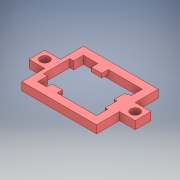
# Autodesk Inventor part: TP4056_long_holder
Saved by Autodesk Inventor 2018 (Build 220112000, 112)
## iProperties
Created: 2019-09-05
Part Number: TP4056_long_holder
Material: Generic
Document SubType Name: Modeling
Designer: ZEUSLAP
Density: 1 g/cm^3
Appearance: Default
Author: ZEUSLAP
## iProperties of the stored document charger_holder_TP4056_3DPrint.ipt
Created: 2019-10-07
Part Number: charger_holder_TP4056_3DPrint
Material: Generic
Document SubType Name: Modeling
Designer: ZEUSLAP
Density: 1 g/cm^3
Appearance: Default
Author: ZEUSLAP
Autodesk Inventor part; units mm, degrees
ref_plane "YZ Plane" through (0, 0, 0) normal (1, 0, 0) x (0, 1, 0)
ref_plane "XZ Plane" through (0, 0, 0) normal (0, 1, 0) x (-1, 0, 0)
ref_plane "XY Plane" through (0, 0, 0) normal (0, 0, 1) x (1, 0, 0)
sketch "shape" plane through (0, 0, 0) normal (0, 0, 1) x (1, 0, 0)
  line L0 (-11.25, 8.75) -> (11.25, 8.75)
  line L1 (11.25, 8.75) -> (11.25, -8.75)
  line L2 (11.25, -8.75) -> (-11.25, -8.75)
  line L3 (-11.25, -8.75) -> (-11.25, 8.75)
  line L4 (14.25, 11.75) -> (-14.25, 11.75)
  line L5 (-14.25, 11.75) -> (-14.25, -11.75)
  line L6 (-14.25, -11.75) -> (14.25, -11.75)
  line L7 (14.25, -11.75) -> (14.25, 11.75)
  line L8 (-12.75, 5) -> (-11.25, 5)
  line L9 (-11.25, 5) -> (-11.25, -5)
  line L10 (-11.25, -5) -> (-12.75, -5)
  line L11 (-12.75, -5) -> (-12.75, 5)
  line L12 (-7.75, -6.75) -> (-3.75, -6.75)
  line L13 (-3.75, -6.75) -> (-3.75, -8.75)
  line L14 (-3.75, -8.75) -> (-7.75, -8.75)
  line L15 (-7.75, -8.75) -> (-7.75, -6.75)
  line L16 (10.25, 4.5) -> (11.25, 4.5)
  line L17 (11.25, 4.5) -> (11.25, -4.5)
  line L18 (11.25, -4.5) -> (10.25, -4.5)
  line L19 (10.25, -4.5) -> (10.25, 4.5)
  line L20 (10.25, 1.5) -> (10.25, -1.5)
  line L21 (-5.75, 8.75) -> (-1.75, 8.75)
  line L22 (-1.75, 8.75) -> (-1.75, 6.25)
  line L23 (-1.75, 6.25) -> (-5.75, 6.25)
  line L24 (-5.75, 6.25) -> (-5.75, 8.75)
  line L25 (-20.25, 3) -> (-14.25, 3)
  line L26 (-14.25, 3) -> (-14.25, -3)
  line L27 (-14.25, -3) -> (-20.25, -3)
  line L28 (-20.25, -3) -> (-20.25, 3)
  line L29 (14.25, 3) -> (20.25, 3)
  line L30 (20.25, 3) -> (20.25, -3)
  line L31 (20.25, -3) -> (14.25, -3)
  line L32 (14.25, -3) -> (14.25, 3)
  circle A0 centre (-17.25, 0) radius 1.75
  circle A1 centre (17.25, 0) radius 1.75
  line L33 (9.25, 4) -> (10.25, 4)
  line L34 (10.25, 4) -> (10.25, 0)
  line L35 (10.25, 0) -> (9.25, 0)
  line L36 (9.25, 0) -> (9.25, 4)
  point P0 (0, 0)
  point P1 (0, 8.75)
  point P2 (11.25, 0)
  point P3 (-12.75, 0)
  point P4 (10.25, 0)
  point P5 (-14.25, 0)
  point P6 (14.25, 0)
  point P7 (-14.25, 0)
  point P8 (14.25, 0)
  point P9 (17.25, 3)
  point P10 (-17.25, 3)
  dimension "d0" = 22.5
  dimension "d1" = 17.5
  dimension "d2" = 3
  dimension "d3" = 1.5
  dimension "d4" = 10
  dimension "d5" = 4
  dimension "d6" = 2
  dimension "d7" = 3.5
  dimension "d8" = 1
  dimension "d9" = 9
  dimension "d12" = 4
  dimension "d13" = 2.5
  dimension "d14" = 13
  dimension "d19" = 6
  dimension "d22" = 3.5
  dimension "d23" = 4
  dimension "d24" = 4.5
  dimension "d25" = 1
  constraints: 74 end point, 18 parallel, 10 midpoint, 9 perpendicular, 8 collinear, 8 horizontal, 7 horizontal alignment, 3 equal length, 3 vertical alignment, 2 centre point, 1 equal radius, 3 other
  measures "d0" distance of L1.end L2.end
  measures "d1" distance of L0.end L1.end
  measures "d2" distance between parallel lines of L0 L4
  measures "d3" distance of L9.end L10.end
  measures "d4" distance of L8.end L9.end
  measures "d5" distance of L13.end L14.end
  measures "d6" distance of L12.end L13.end
  measures "d7" distance between parallel lines of L3 L15
  measures "d8" distance of L17.end L18.end
  measures "d9" distance of L16.end L17.end
  measures "d12" distance of L22.end L23.end
  measures "d13" distance of L21.end L22.end
  measures "d14" distance between parallel lines of L1 L22
  measures "d19" distance of L26.end L27.end
  measures "d22" diameter of A1
  measures "d23" distance of L35.end L33.start
  measures "d24" distance between parallel lines of L18 L35
  measures "d25" distance of L33.start L33.end
extrude "around pcb" add sketch "shape" against normal blind 1.5
extrude "over pcb" add sketch "shape" along normal blind 1.5 contours L0 L22 L23 L24 | L1 L18 L19 L16 | L15 L12 L13 L2 | L19 L35 L36 L33 | L7 L6 L5 L4 | L29 L30 L31 L7 | L5 L27 L28 L25
body "Solid1"
